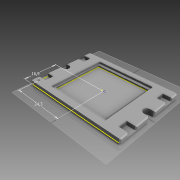
# Autodesk Inventor part: CMV12000
Saved by Autodesk Inventor 2013 (Build 170138000, 138)
## iProperties
Created: 2014-10-21
Part Number: CMV12000
Material: Generic
Document SubType Name: Modeling
Designer: spichelh
Density: 1 g/cm^3
Author: spichelh
Autodesk Inventor part; units mm, degrees
ref_plane "YZ Plane" through (0, 0, 0) normal (1, 0, 0) x (0, 1, 0)
ref_plane "XZ Plane" through (0, 0, 0) normal (0, 1, 0) x (-1, 0, 0)
ref_plane "XY Plane" through (0, 0, 0) normal (0, 0, 1) x (1, 0, 0)
sketch "Sketch2" plane through (0, 0, 0) normal (0, 1, 0) x (-1, 0, 0)
  line L0 (0, 40.0342) -> (0, 27.9116) construction
  line L1 (0, 16.9) -> (-23.5, 16.9)
  line L2 (-23.5, 16.9) -> (-23.5, 12.9)
  line L3 (-23.5, 12.9) -> (-19.5, 12.9)
  line L4 (-19.5, 12.9) -> (-19.5, 8.9)
  line L5 (-19.5, 8.9) -> (-23.5, 8.9)
  line L6 (-23.5, 8.9) -> (-23.5, 1.75)
  line L7 (-23.5, 1.75) -> (-21.5, 1.75)
  line L8 (-21.5, -1.75) -> (-23.5, -1.75)
  line L9 (-23.5, -1.75) -> (-23.5, -8.9)
  line L10 (-23.5, -8.9) -> (-19.5, -8.9)
  line L11 (-19.5, -8.9) -> (-19.5, -12.9)
  line L12 (-19.5, -12.9) -> (-23.5, -12.9)
  line L13 (-23.5, -12.9) -> (-23.5, -16.9)
  line L14 (-23.5, -16.9) -> (0, -16.9)
  line L15 (0, 0) -> (0, 27.9116) construction
  line L16 (0, 0) -> (-32.8795, 0) construction
  line L17 (23.5, -16.9) -> (0, -16.9)
  line L18 (23.5, 16.9) -> (23.5, 12.9)
  line L19 (23.5, 1.75) -> (21.5, 1.75)
  line L20 (23.5, 12.9) -> (19.5, 12.9)
  line L21 (19.5, 12.9) -> (19.5, 8.9)
  line L22 (19.5, 8.9) -> (23.5, 8.9)
  line L23 (21.5, -1.75) -> (23.5, -1.75)
  line L24 (23.5, -1.75) -> (23.5, -8.9)
  line L25 (23.5, -8.9) -> (19.5, -8.9)
  line L26 (19.5, -8.9) -> (19.5, -12.9)
  line L27 (19.5, -12.9) -> (23.5, -12.9)
  line L28 (23.5, -12.9) -> (23.5, -16.9)
  line L29 (23.5, 8.9) -> (23.5, 1.75)
  line L30 (0, 16.9) -> (23.5, 16.9)
  arc A0 (-21.5, -1.75) -> (-21.5, 1.75) centre (-21.5, 0) ccw
  arc A1 (21.5, 1.75) -> (21.5, -1.75) centre (21.5, 0) ccw
  point P0 (0, 0)
  dimension "d33" = 4
  dimension "d34" = 4
  dimension "d35" = 4
  dimension "d36" = 33.8
  dimension "d37" = 4
  dimension "d38" = 3.5
  dimension "d39" = 2
  dimension "d40" = 4
  dimension "d41" = 47
  constraints: 62 end point, 15 symmetric about line, 9 parallel, 8 collinear, 4 point on circle, 3 point on line, 2 centre point, 2 horizontal, 2 perpendicular, 2 tangent, 1 other
  measures "d33" distance of L1.end L2.end
  measures "d34" distance of L3.end L4.end
  measures "d35" distance of L2.end L3.end
  measures "d36" distance between parallel lines of L14 L1
  measures "d37" distance of L12.end L13.end
  measures "d38" distance between parallel lines of L8 L7
  measures "d39" distance of L6.end L7.end
  measures "d40" distance of L10.end L11.end
  measures "d41" distance of L1.end L18.start
extrude "Extrusion1" add sketch "Sketch2" along normal blind 1.75
sketch "Sketch3" plane through (0, 0, 0) normal (0, -1, 0) x (1, 0, 0)
  line L0 (-23.5, 16.9) -> (23.5, 16.9) projected
  line L1 (-23.5, 12.9) -> (-23.5, 16.9) projected
  line L2 (-23.5, 1.75) -> (-23.5, 8.9) projected
  line L3 (-21.5, 1.75) -> (-23.5, 1.75) projected
  arc A0 (-21.5, -1.75) -> (-21.5, 1.75) centre (-21.5, 0) ccw projected
  line L4 (-23.5, -1.75) -> (-21.5, -1.75) projected
  line L5 (-23.5, -8.9) -> (-23.5, -1.75) projected
  line L6 (-23.5, -16.9) -> (-23.5, -12.9) projected
  line L7 (23.5, -16.9) -> (-23.5, -16.9) projected
  line L8 (23.5, -12.9) -> (23.5, -16.9) projected
  line L9 (23.5, -1.75) -> (23.5, -8.9) projected
  line L10 (21.5, -1.75) -> (23.5, -1.75) projected
  arc A1 (21.5, 1.75) -> (21.5, -1.75) centre (21.5, 0) ccw projected
  line L11 (23.5, 1.75) -> (21.5, 1.75) projected
  line L12 (23.5, 8.9) -> (23.5, 1.75) projected
  line L13 (23.5, 16.9) -> (23.5, 12.9) projected
  line L14 (-23.5, -8.9) -> (-23.5, -12.9)
  line L15 (23.5, -12.9) -> (23.5, -8.9)
  line L16 (23.5, 8.9) -> (23.5, 12.9)
  line L17 (-23.5, 8.9) -> (-23.5, 12.9)
  point P0 (0, 0)
  constraints: 8 end point, 2 collinear, 2 parallel
extrude "Extrusion2" add sketch "Sketch3" along normal blind 1
sketch "Sketch4" plane through (0, 1.75, 0) normal (0, 1, 0) x (1, 0, 0)
  line L0 (-23.5, -16.9) -> (23.5, -16.9) projected
  line L1 (-23.5, -12.9) -> (-23.5, -16.9) projected
  circle A0 centre (-21.5, -14.9) radius 0.5
  point P0 (0, 0)
  dimension "d46" = 2
  dimension "d47" = 2
  dimension "d48" = 1
  constraints: 1 centre point, 1 coincident
  measures "d46" distance from line of L0 point (-21.5, -14.9)
  measures "d47" distance from line of L1 point (-21.5, -14.9)
  measures "d48" diameter of A0
extrude "Extrusion3" cut sketch "Sketch4" against normal blind 3
chamfer "Chamfer1" distance 0.5 angle 45 14 edges at (-23.5, 0.375, -16.9) (-23.5, 0.375, 16.9) (23.5, 0.375, 16.9) (23.5, 0.375, -16.9) (23.5, 0.875, 12.9) (23.5, 0.875, 8.9) (23.5, 0.875, -8.9) (23.5, 0.875, -12.9) (23.5, 0.375, 1.75) (23.5, 0.375, -1.75) (-23.5, 0.875, 12.9) (-23.5, 0.875, 8.9) (-23.5, 0.875, -8.9) (-23.5, 0.875, -12.9)
fillet "Fillet1" radius 0.2 8 edges at (-19.5, 0.875, -8.9) (-19.5, 0.875, 8.9) (-19.5, 0.875, 12.9) (-19.5, 0.875, -12.9) (19.5, 0.875, -12.9) (19.5, 0.875, -8.9) (19.5, 0.875, 12.9) (19.5, 0.875, 8.9)
chamfer "Chamfer2" distance 0.5 angle 45 10 edges at (23.5, 1.75, -14.9) (23.5, 1.75, -5.325) (23.5, 1.75, 5.325) (23.5, 1.75, 14.9) (23.5, -1, -9.325) (23.5, -1, 9.325) (-23.5, 1.75, 5.075) (-23.5, 1.75, -5.075) (-23.5, -1, -9.075) (-23.5, -1, 9.075)
sketch "Sketch5" plane through (0, 1.75, 0) normal (0, 1, 0) x (1, 0, 0)
  line L0 (-13.1, 12.4) -> (13.1, 12.4)
  line L1 (13.6, 11.9) -> (13.6, -11.9)
  line L2 (13.1, -12.4) -> (-13.1, -12.4)
  line L3 (-13.6, -11.9) -> (-13.6, 11.9)
  line L4 (-13.6, 12.4) -> (13.6, -12.4) construction
  line L5 (-13.6, -12.4) -> (13.6, 12.4) construction
  arc A0 (-13.1, 12.4) -> (-13.6, 11.9) centre (-13.1, 11.9) ccw
  arc A1 (-13.6, -11.9) -> (-13.1, -12.4) centre (-13.1, -11.9) ccw
  arc A2 (13.1, -12.4) -> (13.6, -11.9) centre (13.1, -11.9) ccw
  arc A3 (13.6, 11.9) -> (13.1, 12.4) centre (13.1, 11.9) ccw
  point P0 (0, 0)
  dimension "d58" = 24.8
  dimension "d60" = 27.2
  dimension "d61" = 0.5
  constraints: 12 end point, 8 point on circle, 8 point on line, 8 tangent, 4 centre point, 3 equal radius, 2 midpoint, 2 parallel, 1 horizontal, 1 perpendicular
  measures "d58" distance between parallel lines of L2 L0
  measures "d60" distance between parallel lines of L3 L1
  measures "d61" radius of A0
extrude "Extrusion4" cut sketch "Sketch5" against normal blind 1.8
sketch "Sketch6" plane through (0, 1.75, 0) normal (0, 1, 0) x (1, 0, 0)
  line L0 (-13.85, 13.9) -> (13.85, 13.9)
  line L1 (14.35, 13.4) -> (14.35, -13.4)
  line L2 (13.85, -13.9) -> (-13.85, -13.9)
  line L3 (-14.35, -13.4) -> (-14.35, 13.4)
  line L4 (14.35, 13.9) -> (-14.35, -13.9) construction
  line L5 (14.35, -13.9) -> (-14.35, 13.9) construction
  arc A0 (-13.6, -11.9) -> (-13.1, -12.4) centre (-13.1, -11.9) ccw projected
  line L6 (-13.6, -11.9) -> (-13.6, 11.9) projected
  arc A1 (-13.1, 12.4) -> (-13.6, 11.9) centre (-13.1, 11.9) ccw projected
  line L7 (-13.1, 12.4) -> (13.1, 12.4) projected
  arc A2 (13.6, 11.9) -> (13.1, 12.4) centre (13.1, 11.9) ccw projected
  line L8 (13.6, 11.9) -> (13.6, -11.9) projected
  arc A3 (13.1, -12.4) -> (13.6, -11.9) centre (13.1, -11.9) ccw projected
  line L9 (13.1, -12.4) -> (-13.1, -12.4) projected
  arc A4 (-13.85, 13.9) -> (-14.35, 13.4) centre (-13.85, 13.4) ccw
  arc A5 (-14.35, -13.4) -> (-13.85, -13.9) centre (-13.85, -13.4) ccw
  arc A6 (13.85, -13.9) -> (14.35, -13.4) centre (13.85, -13.4) ccw
  arc A7 (14.35, 13.4) -> (13.85, 13.9) centre (13.85, 13.4) ccw
  point P0 (0, 0)
  dimension "d64" = 28.7
  dimension "d66" = 27.8
  dimension "d67" = 0.5
  constraints: 12 end point, 8 point on circle, 8 point on line, 8 tangent, 4 centre point, 3 equal radius, 2 midpoint, 2 parallel, 1 horizontal, 1 perpendicular
  measures "d64" distance of L5.end L4.start
  measures "d66" distance of L4.start L5.start
  measures "d67" radius of A4
extrude "Extrusion5" cut sketch "Sketch6" against normal blind 1
sketch "Sketch7" plane through (0, 1.75, 0) normal (0, 1, 0) x (1, 0, 0)
  line L0 (-23, -16.9) -> (23, -16.9) projected
  line L1 (23, 16.9) -> (-23, 16.9) projected
  line L2 (-17.35, 16.9) -> (17.35, 16.9)
  line L3 (17.35, 16.9) -> (17.35, -16.9)
  line L4 (17.35, -16.9) -> (-17.35, -16.9)
  line L5 (-17.35, -16.9) -> (-17.35, 16.9)
  line L6 (17.35, -16.9) -> (-17.35, 16.9) construction
  line L7 (-17.35, -16.9) -> (17.35, 16.9) construction
  point P0 (0, 0)
  dimension "d70" = 34.7
  constraints: 12 end point, 2 parallel, 2 point on line, 1 horizontal, 1 midpoint, 1 perpendicular
  measures "d70" distance between parallel lines of L3 L5
extrude "Extrusion6" [suppressed]
sketch "Sketch8" plane through (0, -0.05, 0) normal (0, 1, 0) x (1, 0, 0)
  line L0 (-13.6, -11.9) -> (-13.6, 11.9) projected
  arc A0 (-13.6, -11.9) -> (-13.1, -12.4) centre (-13.1, -11.9) ccw projected
  line L1 (13.1, -12.4) -> (-13.1, -12.4) projected
  arc A1 (13.1, -12.4) -> (13.6, -11.9) centre (13.1, -11.9) ccw projected
  line L2 (13.6, 11.9) -> (13.6, -11.9) projected
  arc A2 (13.6, 11.9) -> (13.1, 12.4) centre (13.1, 11.9) ccw projected
  line L3 (-13.1, 12.4) -> (13.1, 12.4) projected
  arc A3 (-13.1, 12.4) -> (-13.6, 11.9) centre (-13.1, 11.9) ccw projected
  line L4 (-23.5, -8.4) -> (-23.5, -13.4) projected
  line L5 (-23, -16.9) -> (23, -16.9) projected
  point P0 (0, 0)
  point P1 (0.8, 0)
  dimension "d74" = 24.3
  dimension "d75" = 16.9
  measures "d74" distance from line of L4 point (0.8, 0)
  measures "d75" distance from line of L5 point (0.8, 0)
body "Solid1"
